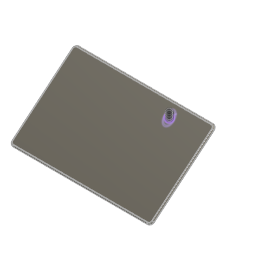
Touchscreen Mount (Autodesk Fusion 360 design; units mm, degrees)
part number: 2026-01-26-22-51-19-411
Autodesk Fusion 360 part; units mm, degrees
sketch "Sketch1" plane through (0, 0, 0) normal (1, 0, 0) x (0, 0, -1)
  line L0 (0, 0) -> (107.1378, 0) construction
  line L1 (107.1378, 0) -> (107.1378, -18) construction
  line L2 (107.1378, -18) -> (0, -18) construction
  line L3 (0, -18) -> (0, 0) construction
  line L4 (0, -18) -> (56.692, -18) construction
  line L5 (56.692, -18) -> (56.692, -63) construction
  line L6 (56.692, -63) -> (0, -63) construction
  line L7 (0, -63) -> (0, -18) construction
  line L8 (0, -63) -> (167.538, -63) construction
  line L9 (167.538, -63) -> (167.538, -143) construction
  line L10 (167.538, -143) -> (0, -143) construction
  line L11 (0, -143) -> (0, -63) construction
  line L12 (0, -83) -> (167.538, -83) construction
  line L13 (0, -114.6161) -> (167.538, -114.6161) construction
  circle A0 centre (-18, -18) radius 18
  line L14 (-81.7571, 91.314) -> (-255.7186, -53.0484)
  line L15 (-255.7186, -53.0484) -> (-250.8525, -58.9123)
  line L16 (-250.8525, -58.9123) -> (-76.8909, 85.4501)
  line L17 (-76.8909, 85.4501) -> (-81.7571, 91.314)
  line L18 (0, 0) -> (0, 100) construction
  circle A1 centre (-18, -18) radius 125.0686 construction
  line L19 (-18, -18) -> (-92.8547, 72.2025) construction
  line L20 (-185.0917, -29.7058) -> (-109.025, 33.4184)
  line L21 (-109.025, 33.4184) -> (-121.4901, 48.4393)
  line L22 (-185.0917, -29.7058) -> (-197.5569, -14.6848)
  line L23 (-3.8835, -6.832) -> (-76.8909, 85.4501)
  line L24 (-31.8517, -29.4948) -> (-106.7064, 60.7076)
  line L25 (-185.0917, -29.7058) -> (-64.7769, 70.1378)
  line L26 (-185.0917, -29.7058) -> (-173.7072, -43.4245)
  line L27 (-173.7072, -43.4245) -> (-82.8567, 31.968)
  dimension "d1" = 18
  dimension "d2" = 45
  dimension "d3" = 80
  dimension "d5" = 20
  dimension "d6" = 31.6161
  dimension "d7" = 7.62
  dimension "d8" = 226.06
  dimension "d9" = 100
  dimension "d10" = 18
  dimension "d11" = 36
  constraint horizontal L0
  constraint vertical L1
  constraint horizontal L2
  constraint vertical L3
  constraint coincident L0.start L3.end
  constraint horizontal L4
  constraint vertical L5
  constraint horizontal L6
  constraint vertical L7
  constraint horizontal L8
  constraint vertical L9
  constraint horizontal L10
  constraint vertical L11
  constraint coincident L11 L12.start
  constraint coincident L9 L12.end
  constraint perpendicular L9 L12
  constraint coincident L11 L13.start
  constraint coincident L9 L13.end
  constraint perpendicular L9 L13
  constraint perpendicular L14 L15
  constraint perpendicular L15 L16
  constraint perpendicular L14 L17
  constraint perpendicular L0 L18
  constraint tangent A0 L18
  constraint concentric A0 A1
  constraint coincident A0.centre A1.centre
  constraint coincident L16 L19.end
  constraint perpendicular L16 L19
  constraint perpendicular L19 L20
  constraint coincident L16 L21.end
  constraint perpendicular L16 L21
  constraint coincident L16 L22.end
  constraint perpendicular L16 L22
  constraint coincident A0 L23.start
  constraint coincident A0 L24.start
  constraint coincident L16 L24.end
  constraint perpendicular L16 L24
  constraint tangent A0 L23
  constraint tangent A0 L24
  constraint coincident L23 L25.end
  constraint perpendicular L19 L25
  constraint perpendicular L25 L26
  constraint coincident L24 L27.end
  constraint perpendicular L24 L27
  measures "d1" distance of L0 L2
  measures "d2" distance of L2 L6
  measures "d3" distance of L6 L10
  measures "d5" distance of L8 L12
  measures "d6" distance of L12 L13
  measures "d7" distance of L14.start L16.end
  measures "d8" distance of L14.start L14.end
  measures "d9" distance of L0.start L18.end
  measures "d10" vertical distance of L0.start A0.centre
  measures "d11" diameter of A0
extrude "Extrude1" add sketch "Sketch1" along normal blind 18 from surface at 60 contours A0 | A0 L23 L24 L25 | L20 L24 L25 L26 L27 makes body 1
fillet "Fillet1" radius 18 1 edges at (69, 70.1378, 64.7769) on bodies 1
fillet "Fillet1" radius 18 1 edges at (69, 31.968, 82.8567) on bodies 1
fillet "Fillet1" radius 9 1 edges at (69, -43.4245, 173.7072) on bodies 1
mirror "Mirror1" about plane through (0, 0, 0) normal (1, 0, 0) of bodies 1 makes body 2
sketch "Sketch2" plane through (0, 73.3679, 60.8845) normal (0, 0.769537, 0.638602) x (1, 0, 0)
  line L0 (-60, -23.4837) -> (-78, -23.4837)
  line L1 (-78, -23.4837) -> (-78, -161.4051)
  line L2 (-78, -161.4051) -> (-60, -161.4051)
  line L3 (-60, -161.4051) -> (-60, -23.4837)
  circle A0 centre (-37.5, -74.7466) radius 2.2
  circle A1 centre (37.5, -74.7466) radius 2.2
  circle A2 centre (37.5, -149.7466) radius 2.2
  circle A3 centre (-37.5, -149.7466) radius 2.2
  line L4 (0, 0) -> (0, -166.9245)
  line L5 (0, -112.2466) -> (84.1795, -112.2466) construction
  circle A4 centre (37.5, -74.7466) radius 6
  circle A5 centre (-37.5, -74.7466) radius 6
  circle A6 centre (-37.5, -149.7466) radius 6
  circle A7 centre (37.5, -149.7466) radius 6
  line L6 (-60, -63.0882) -> (60, -63.0882)
  line L7 (60, -63.0882) -> (60, -161.4051)
  line L8 (60, -161.4051) -> (-60, -161.4051)
  line L9 (-60, -63.0882) -> (-60, -161.4051)
  line L10 (-37.5, -74.7466) -> (-37.5, -63.0882) construction
  line L11 (-37.5, -149.7466) -> (-37.5, -161.4051) construction
  dimension "d23" = 75
  dimension "d24" = 4.4
  dimension "d25" = 12
  dimension "d26" = 75
  constraint equal A0 A3
  constraint equal A1 A3
  constraint equal A1 A2
  constraint coincident L4.start origin
  constraint vertical L4
  constraint coincident L4 L5.start
  constraint perpendicular L4 L5
  constraint symmetric A1 A2 L5
  constraint symmetric A0 A3 L5
  constraint symmetric A2 A3 L4
  constraint concentric A1 A4
  constraint concentric A0 A5
  constraint concentric A3 A6
  constraint concentric A2 A7
  constraint equal A4 A5
  constraint equal A5 A6
  constraint equal A6 A7
  constraint coincident L3 L6.start
  constraint perpendicular L3 L6
  constraint perpendicular L5 L7
  constraint coincident L2.end L3.start
  constraint symmetric L4 L7 L9
  constraint horizontal L8
  constraint coincident A0.centre A5.centre
  constraint coincident L6 L10.end
  constraint perpendicular L6 L10
  constraint coincident A3.centre A6.centre
  constraint coincident L8 L11.end
  constraint perpendicular L8 L11
  constraint equal L10 L11
  measures "d23" distance of A0.centre A1.centre
  measures "d24" diameter of A1
  measures "d25" diameter of A4
  measures "d26" distance of A0.centre A3.centre
extrude "Extrude2" add sketch "Sketch2" against normal blind 8 separate body contours L3 L4 L6 L8 L9 | L4 L6 L7 L8 | A4 | A5 | A6 | A7 makes body 3
extrude "Extrude3" add sketch "Sketch2" against normal up to surface (17.8273 mm away) contours L3 L4 L6 L8 L9 | L4 L6 L7 L8 bodies 3
sketch "Sketch4" plane through (60, 0, 0) normal (1, 0, 0) x (0, 0, -1)
  line L0 (-109.4332, 33.0796) -> (-185.0917, -29.7058)
  line L1 (-185.0917, -29.7058) -> (-173.7072, -43.4245)
  line L2 (-173.7072, -43.4245) -> (-98.0487, 19.3609)
  line L3 (-98.0487, 19.3609) -> (-109.4332, 33.0796)
  circle A0 centre (-112.9754, 18.557) radius 3.6
  circle A1 centre (-141.5702, -5.1724) radius 3.6
  circle A2 centre (-170.165, -28.9019) radius 3.6
  line L4 (-170.165, -28.9019) -> (-179.3995, -36.5651)
  line L5 (-170.165, -28.9019) -> (-141.5702, -5.1724)
  line L6 (-141.5702, -5.1724) -> (-112.9754, 18.557)
  line L7 (-112.9754, 18.557) -> (-103.7409, 26.2203)
  circle A3 centre (-112.9754, 18.557) radius 6.5
  circle A4 centre (-141.5702, -5.1724) radius 6.5
  circle A5 centre (-170.165, -28.9019) radius 6.5
  circle A6 centre (-170.165, -28.9019) radius 3.1
  circle A7 centre (-141.5702, -5.1724) radius 3.1
  circle A8 centre (-112.9754, 18.557) radius 3.1
  dimension "d31" = 7.2
  dimension "d32" = 6.2
  dimension "d33" = 13
  dimension "d34" = 12
  constraint coincident A2.centre L4.start
  constraint midpoint L1 L4.end
  constraint parallel L2 L4
  constraint coincident A1.centre L5.end
  constraint coincident A0.centre L6.end
  constraint collinear L5 L6
  constraint collinear L4 L6
  constraint equal A1 A2
  constraint equal A0 A1
  constraint equal L5 L6
  constraint midpoint L3 L7.end
  constraint equal L4 L7
  constraint concentric A0 A3
  constraint concentric A1 A4
  constraint concentric A2 A5
  constraint concentric A2 A6
  constraint concentric A4 A7
  constraint concentric A0 A8
  constraint equal A7 A8
  constraint equal A6 A7
  constraint equal A4 A5
  constraint equal A3 A5
  measures "d31" diameter of A0
  measures "d32" diameter of A8
  measures "d33" diameter of A3
  measures "d34" distance of L7.end A0.centre
extrude "Extrude4" cut sketch "Sketch4" against normal blind 6 from surface at 18 contours A0 L6 L7 A3 | A0 L6 L7 A3 | A2 L4 L5 A5 | A2 L4 L5 A5 | A0 L6 L7 A8 | A0 L6 L7 A8 | A2 L4 L5 A6 | A2 L4 L5 A6 | L6 L7 A8 | L6 L7 A8 | A1 L5 L6 A4 | A1 L5 L6 A4 | L4 L5 A6 | L4 L5 A6 | A1 L5 L6 A7 | A1 L5 L6 A7 | L5 L6 A7 | L5 L6 A7 bodies 1
extrude "Extrude5" cut sketch "Sketch4" along normal blind 30 contours L6 L7 A8 | L6 L7 A8 | L4 L5 A6 | L4 L5 A6 | L5 L6 A7 | L5 L6 A7 bodies 1
extrude "Extrude6" cut sketch "Sketch4" against normal blind 12 contours A0 L6 L7 A8 | A0 L6 L7 A8 | A2 L4 L5 A6 | A2 L4 L5 A6 | L6 L7 A8 | L6 L7 A8 | L4 L5 A6 | L4 L5 A6 | A1 L5 L6 A7 | A1 L5 L6 A7 | L5 L6 A7 | L5 L6 A7 bodies 3
mirror "Mirror2" about plane through (0, 0, 0) normal (1, 0, 0) of "Extrude6"
sketch "Sketch5" plane through (0, 0, 0) normal (1, 0, 0) x (0, 0, -1)
  line L0 (-36, 0.0986) -> (0, 0.0986)
  line L1 (0, 0.0986) -> (0, -63)
  line L2 (0, -63) -> (-36, -63)
  line L3 (-36, -63) -> (-36, 0.0986)
  circle A0 centre (-18, -18) radius 18
  line L4 (0, -63) -> (167.538, -63)
  constraint horizontal L0
  constraint vertical L1
  constraint horizontal L2
  constraint vertical L3
  constraint coincident L1 origin
  constraint tangent L3 A0
  constraint collinear L2 L4
extrude "Extrude7" add sketch "Sketch1" sketch "Sketch5" along normal up to surface and the other way up to surface separate body contours A0 of sketch 2 contours L0 L1 L3 A0 | L1 L2 L3 A0 end surface through (-60, 0, 0) normal (1, 0, 0) offset -0.4 second end surface through (60, 0, 0) normal (-1, 0, 0) offset -0.4 makes body 4
fillet "Fillet2" radius 18 2 edges at (0, 0.0986, 36) (0, -63, 36) on bodies 4
sketch "Sketch6" plane through (0, 0, 36) normal (0, 0, 1) x (1, 0, 0)
  line L0 (-59.6, -45) -> (59.6, -45)
  line L1 (59.6, -45) -> (59.6, -17.9014)
  line L2 (59.6, -17.9014) -> (-59.6, -17.9014)
  line L3 (-59.6, -17.9014) -> (-59.6, -45)
  circle A0 centre (-40, -40.5) radius 4.2
  circle A1 centre (40, -40.5) radius 4.2
  line L4 (0, 0) -> (0, -75.437)
  circle A2 centre (-40, -40.5) radius 7
  circle A3 centre (40, -40.5) radius 7
  dimension "d50" = 80
  dimension "d51" = 8.4
  dimension "d52" = 14
  dimension "d53" = 14
  dimension "d81" = 40.5
  constraint coincident L4.start origin
  constraint perpendicular L2 L4
  constraint symmetric A0 A1 L4
  constraint concentric A0 A2
  constraint concentric A1 A3
  measures "d51" diameter of A0
  measures "d52" diameter of A2
  measures "d53" diameter of A3
  measures "d81" vertical distance of L4.start A1.centre
extrude "Extrude8" cut sketch "Sketch6" against normal blind 70 contours A0 | A1 bodies 4
extrude "Extrude9" cut sketch "Sketch6" against normal blind 8 contours L0 A2 | L0 A2 | L0 A3 | L0 A3 bodies 4
sketch "Sketch7" plane through (59.6, 0, 0) normal (1, 0, 0) x (0, 0, -1)
  arc A0 (-36, -45) -> (-18, -63) centre (-18, -45) ccw
  line L0 (-18, -63) -> (0, -63)
  line L1 (0, -63) -> (0, 0.0986)
  line L2 (0, 0.0986) -> (-18, 0.0986)
  arc A1 (-18, 0.0986) -> (-36, -17.9014) centre (-18, -17.9014) ccw
  line L3 (-36, -17.9014) -> (-36, -45)
  circle A2 centre (-18, -18) radius 4.2
  arc A3 (-31.8517, -29.4948) -> (-3.8835, -6.832) centre (-18, -18) ccw
  circle A4 centre (-18, -18) radius 15
  circle A5 centre (-18, -18) radius 9.8
  dimension "d58" = 8.4
  dimension "d59" = 30
  dimension "d60" = 19.6
  constraint concentric A2 A3
  constraint concentric A3 A4
  constraint concentric A3 A5
  measures "d58" diameter of A2
  measures "d59" diameter of A4
  measures "d60" diameter of A5
extrude "Extrude10" cut sketch "Sketch7" along normal mid plane 1.6 contours A2 | A4 | A5 bodies 1 4
extrude "Extrude11" cut sketch "Sketch7" against normal blind 136 contours A2 bodies 4
extrude "Extrude12" cut sketch "Sketch7" along normal blind 24 contours A2 bodies 1
extrude "Extrude13" cut sketch "Sketch7" against normal blind 8 from surface at 18.4 contours A5 bodies 1
fillet "Fillet3" radius 9 2 edges at (0, -43.4245, 173.7072) (0, 19.3609, 98.0487) on bodies 3
chamfer "Chamfer1" distance 1 angle 45 18 edges at (78, 24.5441, 83.547) (78, -8.602, 131.7449) (78, -39.7126, 173.362) (78, -33.1022, 182.2732) (78, 14.3327, 132.0239) (78, 62.4215, 65.5854) (78, 24.4278, 28.6141) (78, -31.985, 6.6678) (78, -5.6893, 51.6068) (60, 24.5441, 83.547) (60, -5.6893, 51.6068) (60, -31.985, 6.6678) (60, 24.4278, 28.6141) (60, 62.4215, 65.5854) (60, 14.3327, 132.0239) (60, -33.1022, 182.2732) (60, -39.7126, 173.362) (60, -8.602, 131.7449) on bodies 1
chamfer "Chamfer1" distance 1 angle 45 1 edges at (78, -14.4562, 27.1368) on bodies 1
chamfer "Chamfer2" distance 1 angle 45 14 edges at (59.6, -31.4507, 36) (59.6, -57.7279, 30.7279) (59.6, -63, 9) (59.6, 0.0986, 9) (59.6, -5.1735, 30.7279) (40, -33.5, 36) (40, -47.5, 35.8255) (-40, -33.5, 36) (-40, -47.5, 35.8255) (-59.6, -57.7279, 30.7279) (-59.6, -63, 9) (-59.6, 0.0986, 9) (-59.6, -5.1735, 30.7279) (-59.6, -31.4507, 36) on bodies 4
extrude "Extrude14" add sketch "Sketch1" along normal mid plane 375.92 separate body contours L14 L15 L16 L17 makes body 5
fillet "Fillet4" radius 10 4 edges at (187.96, 88.382, 79.324) (187.96, -55.9804, 253.2856) (-187.96, -55.9804, 253.2856) (-187.96, 88.382, 79.324) on bodies 5
fillet "Fillet5" radius 3.5 16 edges at (0, -53.0484, 255.7186) (-185.0311, -51.178, 253.4647) (-187.96, 19.1328, 168.7379) (-185.0311, 89.4435, 84.011) (0, 91.314, 81.7571) (185.0311, 89.4435, 84.011) (187.96, 19.1328, 168.7379) (185.0311, -51.178, 253.4647) (0, 85.4501, 76.8909) (-185.0311, 83.5797, 79.1449) (-187.96, 13.2689, 163.8717) (-185.0311, -57.0419, 248.5986) (0, -58.9123, 250.8525) (185.0311, -57.0419, 248.5986) (187.96, 13.2689, 163.8717) (185.0311, 83.5797, 79.1449) on bodies 5
mirror "Mirror3" about plane through (0, 0, 0) normal (1, 0, 0) of "Extrude10"
sketch "Sketch8" plane through (0, 0, 0) normal (1, 0, 0) x (0, 0, -1)
  circle A0 centre (-18, -18) radius 18
  line L0 (-17.95, -12.8) -> (-17.95, -9.2)
  arc A1 (-17.95, -9.2) -> (-18.05, -9.2) centre (-18, -9.2) ccw
  line L1 (-18.05, -9.2) -> (-18.05, -12.8)
  arc A2 (-18.05, -12.8) -> (-17.95, -12.8) centre (-18, -12.8) ccw
  line L2 (-18, -12.8) -> (-18, -9.2) construction
  line L3 (-17.95, -7.2) -> (-17.95, -4)
  arc A3 (-17.95, -4) -> (-18.05, -4) centre (-18, -4) ccw
  line L4 (-18.05, -4) -> (-18.05, -7.2)
  arc A4 (-18.05, -7.2) -> (-17.95, -7.2) centre (-18, -7.2) ccw
  line L5 (-18, -7.2) -> (-18, -4) construction
  line L6 (-18, -18) -> (-18, -13.8)
  line L7 (-18, -13.8) -> (-18, -12.8)
  circle A5 centre (-18, -18) radius 4.2
  line L8 (-18, -3) -> (-18, -4)
  circle A6 centre (-18, -18) radius 15
  line L9 (-18, -8.2) -> (-18, -6.564)
  circle A7 centre (-18, -18) radius 9.8
  point P0 (-18, -18)
  dimension "d90" = 0.1
  dimension "d91" = 0.1
  dimension "d92" = 1
  dimension "d93" = 1
  dimension "d94" = 1
  dimension "d95" = 1
  constraint tangent L0 A1
  constraint tangent A1 L1
  constraint parallel L0 L1
  constraint tangent L1 A2
  constraint tangent L0 A2
  constraint tangent L3 A3
  constraint tangent A3 L4
  constraint parallel L3 L4
  constraint tangent L4 A4
  constraint tangent L3 A4
  constraint coincident P0 A0.centre
  constraint vertical L6
  constraint coincident A2.centre L2.start
  constraint parallel L2 L7
  constraint coincident L6.end A5
  constraint vertical L8
  constraint coincident A3.centre L5.end
  constraint coincident L8.start A6
  constraint collinear L5 L6
  constraint vertical L9
  constraint collinear L2 L9
  constraint coincident L9.start A7
  measures "d90" distance of L3 L4
  measures "d91" distance of L0 L1
  measures "d92" distance of A4.centre L9.start
  measures "d93" distance of A3.centre L8.start
  measures "d94" distance of A1.centre L9.start
  measures "d95" distance of A2.centre L6.end
extrude "Extrude15" cut sketch "Sketch8" along normal mid plane 182 contours L0 A1 L1 A2 | L3 A3 L4 A4 bodies 1 2 4
pattern_circular "C-Pattern1" count 6 over 360 about axis through (72.08, -18, 18) along (-1, 0, 0) of "Extrude15"
equation "d81 = 18 mm + 22.5 mm"
